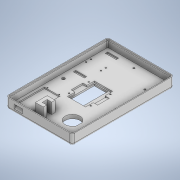
# Autodesk Inventor part: Controller_Front
Saved by Autodesk Inventor 2022.3 (Build 263350000, 350)
## iProperties
Created: 2023-06-20
Part Number: Controller_Front
Material: Generic
Document SubType Name: Modeling
Designer: natalie.jimenez
Density: 1 g/cm^3
Appearance: Default
Author: natalie.jimenez
Autodesk Inventor part; units mm, degrees
ref_plane "YZ Plane" through (0, 0, 0) normal (1, 0, 0) x (0, 1, 0)
ref_plane "XZ Plane" through (0, 0, 0) normal (0, 1, 0) x (-1, 0, 0)
sketch "Sketch1" plane through (0, 0, 0) normal (0, 1, 0) x (-1, 0, 0)
  line L0 (40.64, -63.5) -> (-40.64, -63.5)
  line L1 (-40.64, -63.5) -> (-40.64, 63.5)
  line L2 (-40.64, 63.5) -> (40.64, 63.5)
  line L3 (40.64, 63.5) -> (40.64, -63.5)
  line L4 (40.64, -63.5) -> (-40.64, 63.5) construction
  line L5 (-40.64, -63.5) -> (40.64, 63.5) construction
  point P0 (0, 0)
  dimension "d0" = 127
  dimension "d1" = 81.28
  constraints: 12 end point, 2 midpoint, 2 parallel, 1 horizontal, 1 perpendicular
  measures "d0" distance between parallel lines of L0 L2
  measures "d1" distance between parallel lines of L1 L3
extrude "Extrusion1" add sketch "Sketch1" along normal blind 4.953
sketch "Sketch2" plane through (0, 4.953, 0) normal (0, 1, 0) x (1, 0, 0)
  line L0 (11.7475, 17.4625) -> (-11.7475, 17.4625)
  line L1 (-11.7475, 17.4625) -> (-11.7475, -17.4625)
  line L2 (-11.7475, -17.4625) -> (11.7475, -17.4625)
  line L3 (11.7475, -17.4625) -> (11.7475, 17.4625)
  line L4 (11.7475, 17.4625) -> (-11.7475, -17.4625) construction
  line L5 (-11.7475, 17.4625) -> (11.7475, -17.4625) construction
  point P0 (0, 0)
  dimension "d4" = 23.495
  dimension "d5" = 34.925
  constraints: 12 end point, 2 midpoint, 2 parallel, 1 horizontal, 1 perpendicular
  measures "d4" distance between parallel lines of L3 L1
  measures "d5" distance between parallel lines of L0 L2
extrude "Extrusion2" cut sketch "Sketch2" against normal blind 2.032
sketch "Sketch4" plane through (0, 0, 0) normal (0, 0, 1) x (1, 0, 0)
  line L0 (11.7475, 2.921) -> (17.3304, 4.953)
  line L1 (40.64, 4.953) -> (-40.64, 4.953) projected
  line L2 (11.7475, 4.953) -> (11.7475, 2.921) projected
  line L3 (11.7475, 2.921) -> (11.7475, 4.953)
  line L4 (11.7475, 4.953) -> (17.3304, 4.953)
  point P0 (0, 0)
  dimension "d8" = 70
  constraints: 6 end point, 1 collinear, 1 perpendicular, 1 point on line
  measures "d8" angle of L2 L0
extrude "Extrusion3" cut sketch "Sketch4" along normal mid plane 15.24
sketch "Sketch5" plane through (0, 0, 0) normal (0, 0, 1) x (1, 0, 0)
  line L0 (-11.7475, 2.921) -> (11.7475, 2.921) projected
  line L1 (40.64, 4.953) -> (-40.64, 4.953) projected
  line L2 (-11.7475, 2.921) -> (-16.8275, 2.921)
  line L3 (-16.8275, 2.921) -> (-16.8275, 4.953)
  line L4 (-16.8275, 4.953) -> (-11.7475, 4.953)
  line L5 (-11.7475, 4.953) -> (-11.7475, 2.921)
  point P0 (0, 0)
  point P1 (-11.7475, 3.937)
  point P2 (-16.8275, 3.937)
  point P3 (-11.7475, 4.953)
  dimension "d11" = 5.08
  constraints: 8 end point, 2 midpoint, 2 parallel, 1 horizontal, 1 perpendicular, 1 point on line
  measures "d11" distance of point (-11.748, 3.937) point (-16.828, 3.937)
extrude "Extrusion4" cut sketch "Sketch5" along normal mid plane 15.24
sketch "Sketch6" plane through (0, 2.921, 0) normal (0, 1, 0) x (1, 0, 0)
  line L0 (-11.7475, -17.4625) -> (-11.7475, -7.62) projected
  line L1 (11.7475, -17.4625) -> (-11.7475, -17.4625) projected
  line L2 (11.7475, -7.62) -> (11.7475, -17.4625) projected
  line L3 (11.7475, 7.62) -> (11.7475, -7.62) projected
  line L4 (11.7475, 17.4625) -> (11.7475, 7.62) projected
  line L5 (-11.7475, 17.4625) -> (11.7475, 17.4625) projected
  line L6 (-11.7475, 7.62) -> (-11.7475, 17.4625) projected
  line L7 (-11.7475, 7.62) -> (-16.8275, 7.62) projected
  line L8 (-16.8275, 7.62) -> (-16.8275, -7.62) projected
  line L9 (-16.8275, -7.62) -> (-11.7475, -7.62) projected
  line L10 (-10.6045, 16.0655) -> (6.9215, 16.0655)
  line L11 (6.9215, 16.0655) -> (6.9215, -16.0655)
  line L12 (6.9215, -16.0655) -> (-10.6045, -16.0655)
  line L13 (-10.6045, -16.0655) -> (-10.6045, 16.0655)
  line L14 (11.7475, 7.62) -> (11.7475, -7.62) projected
  line L15 (11.7475, 0) -> (-16.8275, 0) construction
  line L16 (-16.8275, -7.62) -> (-16.8275, 7.62) projected
  line L17 (6.9215, 0) -> (-10.6045, 0) construction
  point P0 (0, 0)
  dimension "d14" = 17.526
  dimension "d15" = 32.131
  dimension "d16" = 4.826
  constraints: 12 end point, 4 midpoint, 2 parallel, 1 collinear, 1 horizontal, 1 perpendicular
  measures "d14" distance between parallel lines of L11 L13
  measures "d15" distance between parallel lines of L12 L10
  measures "d16" distance between parallel lines of L3 L11
extrude "Extrusion5" cut sketch "Sketch6" against normal up to surface (2.921 mm away) contours L10 L11 L12 L13
sketch "Sketch7" plane through (0, 4.953, 0) normal (0, 1, 0) x (1, 0, 0)
  line L0 (-14.2875, 12.7) -> (13.6525, 12.7) construction
  line L1 (13.6525, 12.7) -> (13.6525, -12.7) construction
  line L2 (13.6525, -12.7) -> (-14.2875, -12.7) construction
  line L3 (-14.2875, -12.7) -> (-14.2875, 12.7) construction
  line L4 (-10.6045, -16.0655) -> (-10.6045, 16.0655) projected
  line L5 (-14.2875, 0) -> (13.6525, 0) construction
  line L6 (-10.6045, 0) -> (6.9215, 0) construction
  line L7 (6.9215, 16.0655) -> (6.9215, -16.0655) projected
  line L8 (-11.7475, 7.62) -> (-11.7475, 17.4625) projected
  point P0 (0, 0)
  dimension "d19" = 25.4
  dimension "d20" = 27.94
  dimension "d21" = 2.54
  constraints: 12 end point, 4 midpoint, 3 parallel, 1 collinear, 1 horizontal
  measures "d19" distance of L2.end L0.start
  measures "d20" distance between parallel lines of L1 L3
  measures "d21" distance between parallel lines of L3 L8
hole "Hole1" at (-14.2875, 4.953, -12.7) at (13.6525, 4.953, -12.7) at (13.6525, 4.953, 12.7) at (-14.2875, 4.953, 12.7) direction (0, -1, 0) diameter 1.6942 depth 4.953 thread size "2-56 UNC" class "2B" standard "ANSI Unified Screw Threads"
sketch "Sketch8" plane through (0, 4.953, 0) normal (0, 1, 0) x (1, 0, 0)
  line L0 (-37.1182, -59.7067) -> (-16.7982, -59.7067)
  line L1 (-16.7982, -59.7067) -> (-16.7982, -21.7067)
  line L2 (-16.7982, -21.7067) -> (-37.1182, -21.7067)
  line L3 (-37.1182, -21.7067) -> (-37.1182, -59.7067)
  point P0 (0, 0)
  dimension "d29" = 20.32
  dimension "d30" = 38
  constraints: 8 end point, 2 parallel, 1 horizontal, 1 perpendicular
  measures "d29" distance between parallel lines of L3 L1
  measures "d30" distance between parallel lines of L2 L0
extrude "Extrusion6" cut sketch "Sketch8" against normal blind 1.651
sketch "Sketch11" plane through (0, 4.953, 0) normal (0, 1, 0) x (1, 0, 0)
  line L0 (-34.5782, -61.0275) -> (-19.3382, -61.0275) construction
  line L1 (-16.7982, -59.7067) -> (-37.1182, -59.7067) projected
  line L2 (-19.3382, -61.0275) -> (-19.3382, -20.3875) construction
  line L3 (-19.3382, -20.3875) -> (-34.5782, -20.3875) construction
  line L4 (-34.5782, -20.3875) -> (-34.5782, -61.0275) construction
  line L5 (-37.1182, -21.7067) -> (-16.7982, -21.7067) projected
  line L6 (-37.1182, -59.7067) -> (-37.1182, -21.7067) projected
  line L7 (-16.7982, -21.7067) -> (-16.7982, -59.7067) projected
  line L8 (-16.7982, -59.7067) -> (-37.1182, -59.7067) projected
  line L9 (-16.7982, -21.7067) -> (-16.7982, -59.7067) projected
  line L10 (-37.1182, -21.7067) -> (-16.7982, -21.7067) projected
  line L11 (-37.1182, -59.7067) -> (-37.1182, -21.7067) projected
  line L12 (-16.7982, -59.7067) -> (-37.1182, -59.7067) projected
  line L13 (-34.5782, -40.7075) -> (-37.1182, -40.7067)
  line L14 (-37.1182, -59.7067) -> (-37.1182, -21.7067) projected
  line L15 (-19.3382, -40.7075) -> (-16.7982, -40.7067)
  line L16 (-16.7982, -21.7067) -> (-16.7982, -59.7067) projected
  point P0 (0, 0)
  dimension "d38" = 15.24
  dimension "d39" = 40.64
  dimension "d40" = 1.3208
  constraints: 12 end point, 5 parallel, 4 midpoint, 3 perpendicular, 1 equal length
  measures "d38" distance from line of L0.end L4
  measures "d39" distance between parallel lines of L3 L0
  measures "d40" distance between parallel lines of L1 L0
hole "Hole2" at (-34.5782, 4.953, 20.3875) at (-19.3382, 4.953, 20.3875) at (-19.3382, 4.953, 61.0275) at (-34.5782, 4.953, 61.0275) direction (0, -1, 0) diameter 1.3835 depth 4.953 thread size "M1.6x0.2" class "6H" standard "ANSI Metric M Profile"
sketch "Sketch12" plane through (0, 4.953, 0) normal (0, 1, 0) x (1, 0, 0)
  line L0 (-7.747, 38.227) -> (37.719, 38.227) construction
  line L1 (37.719, 38.227) -> (37.719, 59.309) construction
  line L2 (37.719, 59.309) -> (-7.747, 59.309) construction
  line L3 (-7.747, 59.309) -> (-7.747, 38.227) construction
  line L4 (-0.508, 57.15) -> (30.48, 57.15) construction
  line L5 (30.48, 57.15) -> (30.48, 40.386) construction
  line L6 (30.48, 40.386) -> (-0.508, 40.386) construction
  line L7 (-0.508, 40.386) -> (-0.508, 57.15) construction
  line L8 (-40.64, -63.5) -> (40.64, -63.5) projected
  line L9 (40.64, -63.5) -> (40.64, 63.5) projected
  line L10 (-0.508, 48.768) -> (-7.747, 48.768) construction
  line L11 (30.48, 48.768) -> (37.719, 48.768) construction
  line L12 (40.64, 63.5) -> (-40.64, 63.5) projected
  point P0 (0, 0)
  dimension "d49" = 21.082
  dimension "d63" = 16.764
  dimension "d64" = 30.988
  dimension "d114" = 6.35
  dimension "d115" = 10.16
  constraints: 20 end point, 4 midpoint, 4 parallel, 3 perpendicular, 2 horizontal, 1 collinear
  measures "d49" distance between parallel lines of L2 L0
  measures "d63" distance between parallel lines of L4 L6
  measures "d64" distance between parallel lines of L5 L7
  measures "d114" distance between parallel lines of L12 L4
  measures "d115" distance between parallel lines of L9 L5
hole "Hole3" at (-0.508, 4.953, -57.15) at (30.48, 4.953, -40.386) direction (0, -1, 0) diameter 2.1565 depth 4.953 thread size "4-40 UNC" class "2B" standard "ANSI Unified Screw Threads"
sketch "Sketch13" plane through (0, 4.953, 0) normal (0, 1, 0) x (1, 0, 0)
  circle A0 centre (18.161, -40.64) radius 9.525
  line L0 (40.64, -63.5) -> (40.64, 63.5) projected
  line L1 (40.64, 63.5) -> (-40.64, 63.5) projected
  line L2 (26.924, -44.373) -> (26.924, -36.907)
  line L3 (8.636, -40.64) -> (26.924, -40.64) construction
  line L4 (-40.64, -63.5) -> (40.64, -63.5) projected
  point P0 (0, 0)
  point P1 (17.78, -40.64)
  dimension "d65" = 19.05
  dimension "d98" = 18.288
  dimension "d116" = 22.86
  dimension "d117" = 22.86
  constraints: 4 end point, 3 point on circle, 2 midpoint, 1 centre point, 1 vertical
  measures "d65" diameter of A0
  measures "d98" distance of L3.start L3.end
  measures "d116" distance from line of L4 point (17.78, -40.64)
  measures "d117" distance from line of L0 point (17.78, -40.64)
extrude "Extrusion7" cut sketch "Sketch13" against normal up to surface (4.953 mm away) contours L2 A0 picked at (20.828, -40.64)
sketch "Sketch14" plane through (0, 4.953, 0) normal (0, 1, 0) x (1, 0, 0)
  line L0 (-35.56, 58.42) -> (-21.463, 58.42) construction
  line L1 (-21.463, 58.42) -> (-21.463, 13.97) construction
  line L2 (-21.463, 13.97) -> (-35.56, 13.97) construction
  line L3 (-35.56, 13.97) -> (-35.56, 58.42) construction
  line L4 (-35.56, 13.97) -> (-21.463, 13.97)
  line L5 (-21.463, 13.97) -> (-21.463, 17.145)
  line L6 (-21.463, 17.145) -> (-35.56, 17.145)
  line L7 (-35.56, 17.145) -> (-35.56, 13.97)
  line L8 (-35.56, 58.42) -> (-21.463, 58.42)
  line L9 (-21.463, 58.42) -> (-21.463, 55.245)
  line L10 (-21.463, 55.245) -> (-35.56, 55.245)
  line L11 (-35.56, 55.245) -> (-35.56, 58.42)
  line L12 (-40.64, 63.5) -> (-40.64, -63.5) projected
  line L13 (40.64, 63.5) -> (-40.64, 63.5) projected
  point P0 (0, 0)
  point P1 (-35.56, 15.5575)
  point P2 (-28.5115, 58.42)
  dimension "d72" = 44.45
  dimension "d73" = 14.097
  dimension "d74" = 3.175
  dimension "d75" = 3.175
  dimension "d76" = 5.08
  dimension "d77" = 5.08
  constraints: 24 end point, 6 parallel, 3 horizontal, 3 perpendicular, 2 midpoint, 2 point on line
  measures "d72" distance between parallel lines of L2 L0
  measures "d73" distance between parallel lines of L3 L1
  measures "d74" distance between parallel lines of L6 L2
  measures "d75" distance between parallel lines of L0 L10
  measures "d76" distance from line of L12 point (-35.56, 15.557)
  measures "d77" distance from line of L13 point (-28.512, 58.42)
extrude "Extrusion8" cut sketch "Sketch14" against normal blind 1.524
sketch "Sketch15" plane through (0, 4.953, 0) normal (0, 1, 0) x (1, 0, 0)
  line L0 (-35.56, 13.97) -> (-35.56, 17.145) projected
  line L1 (-35.56, 58.42) -> (-21.463, 58.42) construction
  line L2 (-35.56, 13.97) -> (-21.463, 13.97)
  line L3 (-21.463, 13.97) -> (-21.463, 58.42) construction
  line L4 (-21.463, 58.42) -> (-35.56, 58.42)
  line L5 (-35.56, 58.42) -> (-35.56, 13.97) construction
  line L6 (-38.1, 33.02) -> (-18.923, 33.02) construction
  line L7 (-18.923, 39.37) -> (-38.1, 39.37) construction
  line L8 (-21.463, 55.245) -> (-35.56, 55.245) projected
  line L9 (-35.56, 17.145) -> (-21.463, 17.145) projected
  line L10 (-28.5115, 17.145) -> (-28.5115, 33.02) construction
  line L11 (-28.5115, 39.37) -> (-28.5115, 55.245) construction
  point P0 (0, 0)
  point P1 (-38.1, 39.37)
  dimension "d85" = 6.35
  dimension "d86" = 6.35
  dimension "d89" = 19.05
  dimension "d90" = 19.05
  dimension "d118" = 2.54
  dimension "d119" = 2.54
  dimension "d120" = 2.54
  constraints: 16 end point, 4 midpoint, 3 parallel, 2 horizontal, 1 coincident, 1 equal length, 1 perpendicular
  measures "d85" distance of point (-38.1, 39.37) L6.start
  measures "d86" distance of L7.start L6.end
  measures "d89" distance between parallel lines of L1 L7
  measures "d90" distance between parallel lines of L2 L6
  measures "d118" distance from line of L6.start L5
  measures "d119" distance from line of point (-38.1, 39.37) L5
  measures "d120" distance from line of L3 L6.end
hole "Hole4" at (-38.1, 4.953, -33.02) at (-38.1, 4.953, -39.37) at (-18.923, 4.953, -39.37) at (-18.923, 4.953, -33.02) direction (0, -1, 0) diameter 1.6942 depth 4.953 thread size "2-56 UNC" class "3B" standard "ANSI Unified Screw Threads"
sketch "Sketch16" plane through (0, 0, 0) normal (0, -1, 0) x (1, 0, 0)
  line L0 (-42.672, -65.532) -> (42.672, -65.532)
  line L1 (42.672, -65.532) -> (42.672, 65.532)
  line L2 (42.672, 65.532) -> (-42.672, 65.532)
  line L3 (-42.672, 65.532) -> (-42.672, -65.532)
  line L4 (40.64, -63.5) -> (-40.64, -63.5) projected
  line L5 (-40.64, 63.5) -> (40.64, 63.5) projected
  line L6 (-40.64, -63.5) -> (-40.64, 63.5) projected
  line L7 (40.64, 63.5) -> (40.64, -63.5) projected
  point P0 (0, 0)
  dimension "d99" = 2.032
  dimension "d100" = 2.032
  dimension "d101" = 2.032
  dimension "d102" = 2.032
  constraints: 8 end point, 2 parallel, 1 horizontal, 1 perpendicular
  measures "d99" distance between parallel lines of L4 L0
  measures "d100" distance between parallel lines of L2 L5
  measures "d101" distance between parallel lines of L3 L6
  measures "d102" distance between parallel lines of L1 L7
extrude "Extrusion9" add sketch "Sketch16" against normal blind 12.7
sketch "Sketch17" plane through (-42.672, 0, 65.532) normal (0, 0, 1) x (1, 0, 0)
  line L0 (25.8738, 4.953) -> (5.5538, 4.953) construction
  line L1 (21.209, 4.953) -> (7.112, 4.953) projected
  line L2 (83.312, 12.7) -> (2.032, 12.7) projected
  line L3 (12.8022, 4.953) -> (10.2528, 4.953)
  line L4 (10.2528, 4.953) -> (10.2528, 10.287)
  line L5 (12.8022, 4.953) -> (21.1748, 4.953)
  line L6 (21.1748, 4.953) -> (21.1748, 10.287)
  line L7 (21.209, 4.953) -> (7.112, 4.953) projected
  line L8 (10.2528, 10.287) -> (21.1748, 10.287)
  line L9 (5.5538, 4.953) -> (10.2528, 10.287) construction
  line L10 (5.5538, 4.953) -> (25.8738, 4.953) projected
  line L11 (21.1748, 10.287) -> (25.8738, 4.953) construction
  line L12 (25.8738, 3.302) -> (5.5538, 3.302) projected
  line L13 (85.344, 0) -> (0, 0) projected
  line L14 (85.344, 0) -> (85.344, 12.7) projected
  line L15 (0, 12.7) -> (85.344, 12.7) projected
  line L16 (0, 0) -> (0, 12.7) projected
  line L17 (21.1748, 10.287) -> (21.1748, 4.953)
  point P0 (42.672, 0)
  point P1 (11.5275, 4.953)
  point P2 (10.2528, 7.62)
  point P3 (10.2528, 4.953)
  point P4 (21.1748, 4.953)
  dimension "d109" = 10.922
  dimension "d110" = 5.334
  constraints: 16 end point, 5 perpendicular, 2 equal length, 2 horizontal, 2 midpoint, 1 point on line
  measures "d109" distance of L4.end L6.end
  measures "d110" distance between parallel lines of L8 L0
extrude "Extrusion10" cut sketch "Sketch17" against normal up to surface (2.032 mm away) contours L1 L4 L8 L6
fillet "Fillet1" radius 3.175 8 edges at (-42.672, 0, 0) (0, 0, 65.532) (42.672, 0, 0) (0, 0, -65.532) (-42.672, 6.35, -65.532) (42.672, 6.35, -65.532) (-42.672, 6.35, 65.532) (42.672, 6.35, 65.532)
fillet "Fillet2" radius 1.143 4 edges at (-40.64, 8.8265, 63.5) (-40.64, 8.8265, -63.5) (40.64, 8.8265, 63.5) (40.64, 8.8265, -63.5)
sketch "Sketch18" plane through (0, 12.7, 0) normal (0, 1, 0) x (1, 0, 0)
  line L0 (-39.497, -65.532) -> (39.497, -65.532) projected
  arc A0 (-42.672, -62.357) -> (-39.497, -65.532) centre (-39.497, -62.357) ccw projected
  line L1 (-42.672, 62.357) -> (-42.672, -62.357) projected
  arc A1 (-39.497, 65.532) -> (-42.672, 62.357) centre (-39.497, 62.357) ccw projected
  line L2 (39.497, 65.532) -> (-39.497, 65.532) projected
  arc A2 (42.672, 62.357) -> (39.497, 65.532) centre (39.497, 62.357) ccw projected
  line L3 (42.672, -62.357) -> (42.672, 62.357) projected
  arc A3 (39.497, -65.532) -> (42.672, -62.357) centre (39.497, -62.357) ccw projected
  arc A4 (-41.656, -62.357) -> (-39.497, -64.516) centre (-39.497, -62.357) ccw
  line L4 (-39.497, -64.516) -> (39.497, -64.516)
  arc A5 (39.497, -64.516) -> (41.656, -62.357) centre (39.497, -62.357) ccw
  line L5 (41.656, -62.357) -> (41.656, 62.357)
  arc A6 (41.656, 62.357) -> (39.497, 64.516) centre (39.497, 62.357) ccw
  line L6 (39.497, 64.516) -> (-39.497, 64.516)
  arc A7 (-39.497, 64.516) -> (-41.656, 62.357) centre (-39.497, 62.357) ccw
  line L7 (-41.656, 62.357) -> (-41.656, -62.357)
  point P0 (0, 0)
  dimension "d123" = 1.016
  constraints: 8 end point, 8 point on circle, 4 centre point, 7 other
  measures "d123" distance between parallel lines of L1 L7
extrude "Extrusion11" add sketch "Sketch18" along normal blind 1.27
sketch "Sketch20" plane through (0, 4.953, 0) normal (0, 1, 0) x (1, 0, 0)
  arc A0 (-1.7695, -59.817) -> (-1.7695, -62.357) centre (-1.7695, -61.087) ccw projected
  arc A1 (-1.7695, -59.817) -> (-0.4995, -58.547) centre (-1.7695, -58.547) ccw projected
  line L0 (-0.4995, -54.102) -> (-0.4995, -58.547) projected
  arc A2 (-0.4995, -54.102) -> (-1.7695, -52.832) centre (-1.7695, -54.102) ccw projected
  line L1 (-4.9445, -52.832) -> (-1.7695, -52.832) projected
  arc A3 (-6.2145, -51.562) -> (-4.9445, -52.832) centre (-4.9445, -51.562) ccw projected
  line L2 (-6.2145, -50.292) -> (-6.2145, -51.562) projected
  arc A4 (-4.9445, -49.022) -> (-6.2145, -50.292) centre (-4.9445, -50.292) ccw projected
  line L3 (-1.7695, -49.022) -> (-4.9445, -49.022) projected
  arc A5 (-1.7695, -49.022) -> (-0.4995, -47.752) centre (-1.7695, -47.752) ccw projected
  line L4 (-0.4995, -43.307) -> (-0.4995, -47.752) projected
  arc A6 (-0.4995, -43.307) -> (-1.7695, -42.037) centre (-1.7695, -43.307) ccw projected
  arc A7 (-1.7695, -39.497) -> (-1.7695, -42.037) centre (-1.7695, -40.767) ccw projected
  line L5 (0.7705, -39.497) -> (-1.7695, -39.497) projected
  arc A8 (2.0405, -40.767) -> (0.7705, -39.497) centre (0.7705, -40.767) ccw projected
  line L6 (2.0405, -61.087) -> (2.0405, -40.767) projected
  arc A9 (0.7705, -62.357) -> (2.0405, -61.087) centre (0.7705, -61.087) ccw projected
  line L7 (-1.7695, -62.357) -> (0.7705, -62.357) projected
  arc A10 (-11.2945, -62.357) -> (-11.2945, -59.817) centre (-11.2945, -61.087) ccw projected
  line L8 (-14.4695, -62.357) -> (-11.2945, -62.357) projected
  arc A11 (-15.7395, -61.087) -> (-14.4695, -62.357) centre (-14.4695, -61.087) ccw projected
  line L9 (-15.7395, -40.767) -> (-15.7395, -61.087) projected
  arc A12 (-14.4695, -39.497) -> (-15.7395, -40.767) centre (-14.4695, -40.767) ccw projected
  line L10 (-11.2945, -39.497) -> (-14.4695, -39.497) projected
  arc A13 (-11.2945, -42.037) -> (-11.2945, -39.497) centre (-11.2945, -40.767) ccw projected
  line L11 (-11.9295, -42.037) -> (-11.2945, -42.037) projected
  arc A14 (-11.9295, -42.037) -> (-13.1995, -43.307) centre (-11.9295, -43.307) ccw projected
  line L12 (-13.1995, -58.547) -> (-13.1995, -43.307) projected
  arc A15 (-13.1995, -58.547) -> (-11.9295, -59.817) centre (-11.9295, -58.547) ccw projected
  line L13 (-11.2945, -59.817) -> (-11.9295, -59.817) projected
  line L14 (-11.9295, -58.547) -> (-1.7695, -58.547)
  line L15 (-1.7695, -58.547) -> (-1.7695, -54.102)
  line L16 (-1.7695, -54.102) -> (-7.4845, -54.102)
  line L17 (-7.4845, -54.102) -> (-7.4845, -47.752)
  line L18 (-7.4845, -47.752) -> (-1.7695, -47.752)
  line L19 (-1.7695, -47.752) -> (-1.7695, -43.307)
  line L20 (-1.7695, -43.307) -> (-11.9295, -43.307)
  line L21 (-11.9295, -43.307) -> (-11.9295, -58.547)
  point P0 (0, 0)
  dimension "d133" = 4.445
  dimension "d134" = 4.445
  constraints: 16 end point, 8 perpendicular, 1 horizontal
  measures "d133" distance between parallel lines of L16 L14
  measures "d134" distance between parallel lines of L21 L17
ref_plane "Work Plane1" through (-15.6845, 12.7, 39.497) normal (0, -1, 0) x (1, 0, 0)
extrude "Extrusion12" add sketch "Sketch20" along normal blind 13.8684 contours L21 L20 L19 L18 L17 L16 L15 L14
sketch "Sketch19" plane through (0, 0, 0) normal (0, -1, 0) x (1, 0, 0)
  circle A0 centre (-34.29, 0) radius 1.905 projected
  circle A1 centre (34.29, 0) radius 1.905 projected
  point P0 (0, 0)
hole "Hole5" at (34.29, 0, 0) at (-34.29, 0, 0) direction (0, 1, 0) diameter 3.81 depth 4.953 countersink diameter 7.0866 countersink angle 82 clearance for "Flat Head Machine Screw (82)" size "#6" standard "Ansi Unified Screw Threads"
chamfer "Chamfer1" distance 2.032 angle 20 4 edges at (6.9215, 0, 0) (-1.8415, 0, 16.0655) (-1.8415, 0, -16.0655) (-10.6045, 0, 0) measured on face at (-9.9031, 0, 40.685)
equation "\"d134\" = d133"
body "Solid1"
